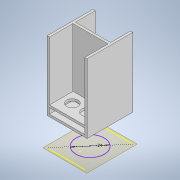
# Autodesk Inventor part: Tclamp_enclosure
Saved by Autodesk Inventor 2022 (Build 260153000, 153)
## iProperties
Created: 2022-06-07
Part Number: Tclamp_enclosure
Material: Generic
Document SubType Name: Modeling
Designer: tecware
Density: 1 g/cm^3
Appearance: Default
Author: tecware
## iProperties of the stored document Tclamp_enclosure_3DPrint.ipt
Created: 2022-06-07
Part Number: Tclamp_enclosure_3DPrint
Material: Generic
Document SubType Name: Modeling
Designer: tecware
Density: 1 g/cm^3
Appearance: Default
Author: tecware
Autodesk Inventor part; units mm, degrees
ref_plane "YZ Plane" through (0, 0, 0) normal (1, 0, 0) x (0, 1, 0)
ref_plane "XY Plane" through (0, 0, 0) normal (0, 0, 1) x (1, 0, 0)
ref_plane "bottom of connector plate" through (0, -2, 0) normal (0, 1, 0) x (-1, 0, 0)
sketch "Sketch1" plane through (0, 0, 0) normal (0, 1, 0) x (-1, 0, 0)
  line L0 (17, -11) -> (-17, -11)
  line L1 (-17, -11) -> (-17, 11)
  line L2 (-17, 11) -> (17, 11)
  line L3 (17, 11) -> (17, -11)
  line L4 (17, -11) -> (-17, 11) construction
  line L5 (-17, -11) -> (17, 11) construction
  line L6 (15, -9) -> (-15, -9)
  line L7 (-15, -9) -> (-15, 9)
  line L8 (-15, 9) -> (15, 9)
  line L9 (15, 9) -> (15, -9)
  line L10 (15, -9) -> (-15, 9) construction
  line L11 (-15, -9) -> (15, 9) construction
  line L12 (17, -11) -> (-17, -11)
  line L13 (-17, -11) -> (-17, -28)
  line L14 (-17, -28) -> (17, -28)
  line L15 (17, -28) -> (17, -11)
  line L16 (15, -11) -> (-15, -11)
  line L17 (-15, -11) -> (-15, -26)
  line L18 (-15, -26) -> (15, -26)
  line L19 (15, -26) -> (15, -11)
  line L20 (15, 9) -> (15, 11)
  line L21 (-15, 9) -> (-15, 11)
  line L22 (-15, -26) -> (-15, -28)
  line L23 (15, -26) -> (15, -28)
  line L24 (15, -9) -> (17, -9)
  line L25 (-15, -9) -> (-17, -9)
  point P0 (0, 0)
  dimension "d0" = 34
  dimension "d1" = 22
  dimension "d2" = 30
  dimension "d3" = 18
  dimension "d5" = 17
  dimension "d6" = 15
  constraints: 52 end point, 10 point on line, 4 midpoint
  measures "d0" distance of L1.end L2.end
  measures "d1" distance of L0.end L1.end
  measures "d2" distance of L7.end L8.end
  measures "d3" distance of L6.end L7.end
  measures "d5" distance of L13.end L12.end
  measures "d6" distance of L17.end L16.end
extrude "top" add sketch "Sketch1" along normal blind 50 contours L15 L14 L23 L19 L0 | L0 L1 L25 L6 L24 L3 | L24 L9 L20 L2 L3 | L17 L22 L14 L13 L0 | L25 L1 L2 L21 L7
sketch "Sketch2" plane through (0, 0, 0) normal (0, 1, 0) x (-1, 0, 0)
  line L0 (17, -28) -> (17, 11) projected
  line L1 (-17, 11) -> (-17, -28) projected
  line L2 (17, 11) -> (-17, 11)
  line L3 (-17, 11) -> (-17, -28)
  line L4 (-17, -28) -> (17, -28)
  line L5 (17, -28) -> (17, 11)
  line L6 (-15, -11) -> (15, -11)
  line L7 (15, -26) -> (-15, -26)
  line L8 (15, -11) -> (-15, -11)
  line L9 (-15, -11) -> (-15, -26)
  line L10 (-15, -26) -> (15, -26)
  line L11 (15, -26) -> (15, -11)
  line L12 (15, 11) -> (15, -9)
  line L13 (-15, -9) -> (-15, 11)
  line L14 (15, -9) -> (-15, -9)
  line L15 (-15, -9) -> (-15, 11)
  line L16 (-15, 11) -> (15, 11)
  line L17 (15, 11) -> (15, -9)
  circle A0 centre (6.5, 0) radius 4.8
  circle A1 centre (-6.5, 0.1042) radius 4.8
  line L18 (6.5, 0) -> (0, 0) construction
  line L19 (-15, -26) -> (-15, -28)
  line L20 (15, -26) -> (15, -28)
  point P0 (17, -9)
  point P1 (-17, -9)
  dimension "d10" = 9.6
  dimension "d11" = 9.6
  dimension "d12" = 13
  dimension "d13" = 6.5
  constraints: 38 end point, 2 centre point, 2 point on line
  measures "d10" diameter of A0
  measures "d11" diameter of A1
  measures "d12" horizontal distance of A1.centre L18.start
  measures "d13" distance of L18.start L18.end
extrude "plate" add sketch "Sketch2" against normal blind 2 contours L4 L20 L11 L6 L9 L19 L1 L2 L13 L14 L12 L0 | L12 L14 L13 L2
sketch "Sketch3" plane through (0, -2, 0) normal (0, 1, 0) x (-1, 0, 0)
  line L0 (17, 11) -> (17, -28)
  line L1 (17, -28) -> (-17, -28)
  line L2 (17, 11) -> (-17, 11)
  line L3 (-17, 11) -> (-17, -28)
  line L4 (-17, -28) -> (17, -28)
  line L5 (17, -28) -> (17, 11)
  line L6 (-15, -26) -> (15, -26)
  line L7 (15, 11) -> (15, -9)
  line L8 (-15, -26) -> (15, -26)
  line L9 (15, -26) -> (15, 9)
  line L10 (15, 9) -> (-15, 9)
  line L11 (-15, 9) -> (-15, -26)
  line L12 (15, 11) -> (15, -9)
  line L13 (15, 9) -> (15, 11)
  line L14 (-15, -9) -> (-15, 11)
  line L15 (-15, 9) -> (-15, 11)
  line L16 (-15, -11) -> (15, -11) projected
  line L17 (17, -9) -> (-17, -9)
  line L18 (15, -11) -> (-15, -11)
  line L19 (-15, -11) -> (-15, -9)
  line L20 (-15, -9) -> (15, -9)
  line L21 (15, -9) -> (15, -11)
  line L22 (-15, -26) -> (-15, -28)
  line L23 (15, -26) -> (15, -28)
  point P0 (0, 0)
  point P1 (15, -26)
  dimension "d17" = 35
  constraints: 46 end point, 3 point on line
  measures "d17" distance of L9.end L8.end
extrude "base" add sketch "Sketch3" against normal blind 4.75 contours L0 L17 L7 L2 | L0 L1 L23 L9 L17 | L9 L16 L11 L17 | L14 L11 L17 L3 L2 | L11 L22 L1 L3 L17
sketch "Sketch6" plane through (-15, -8.75, -9) normal (0, 0, 1) x (1, 0, 0)
  line L0 (30, 2) -> (30, 58.75) projected
  line L1 (30, 2) -> (27, 2)
  line L2 (27, 2) -> (27, 5)
  line L3 (27, 5) -> (30, 5)
  line L4 (30, 5) -> (30, 2)
  line L5 (16.5, 5) -> (16.5, 2)
  line L6 (13.5, 5) -> (13.5, 2)
  line L7 (13.5, 5) -> (16.5, 5)
  line L8 (16.5, 2) -> (13.5, 2)
  point P0 (15, 8.75)
  dimension "d23" = 3
  dimension "d24" = 3
  constraints: 16 end point
  measures "d23" distance of L2.end L3.end
  measures "d24" distance of L1.end L2.end
extrude "Extrusion4" cut sketch "Sketch6" against normal blind 2
sketch "Sketch5" plane through (0, -6.75, 0) normal (0, 1, 0) x (-1, 0, 0)
  line L0 (-17, -28) -> (17, -28)
  line L1 (17, 11) -> (-17, 11)
  line L2 (-17, 11) -> (-17, -28)
  line L3 (-17, -28) -> (17, -28)
  line L4 (17, -28) -> (17, 11)
  constraints: 10 end point
extrude "Extrusion5" add sketch "Sketch5" against normal blind 2
ref_plane "Work Plane4" through (0, -32.5, 0) normal (0, 1, 0) x (-1, 0, 0)
sketch "Sketch4" plane through (0, -32.5, 0) normal (0, 1, 0) x (-1, 0, 0)
  line L0 (-15, 11) -> (15, 11) projected
  line L1 (-17, -28) -> (17, -28) projected
  line L2 (17, 11) -> (-17, -28) construction
  circle A0 centre (0, -8.5) radius 12
  point P0 (0, 0)
  dimension "d22" = 24
  constraints: 2 end point, 1 centre point
  measures "d22" diameter of A0
body "Solid1"
